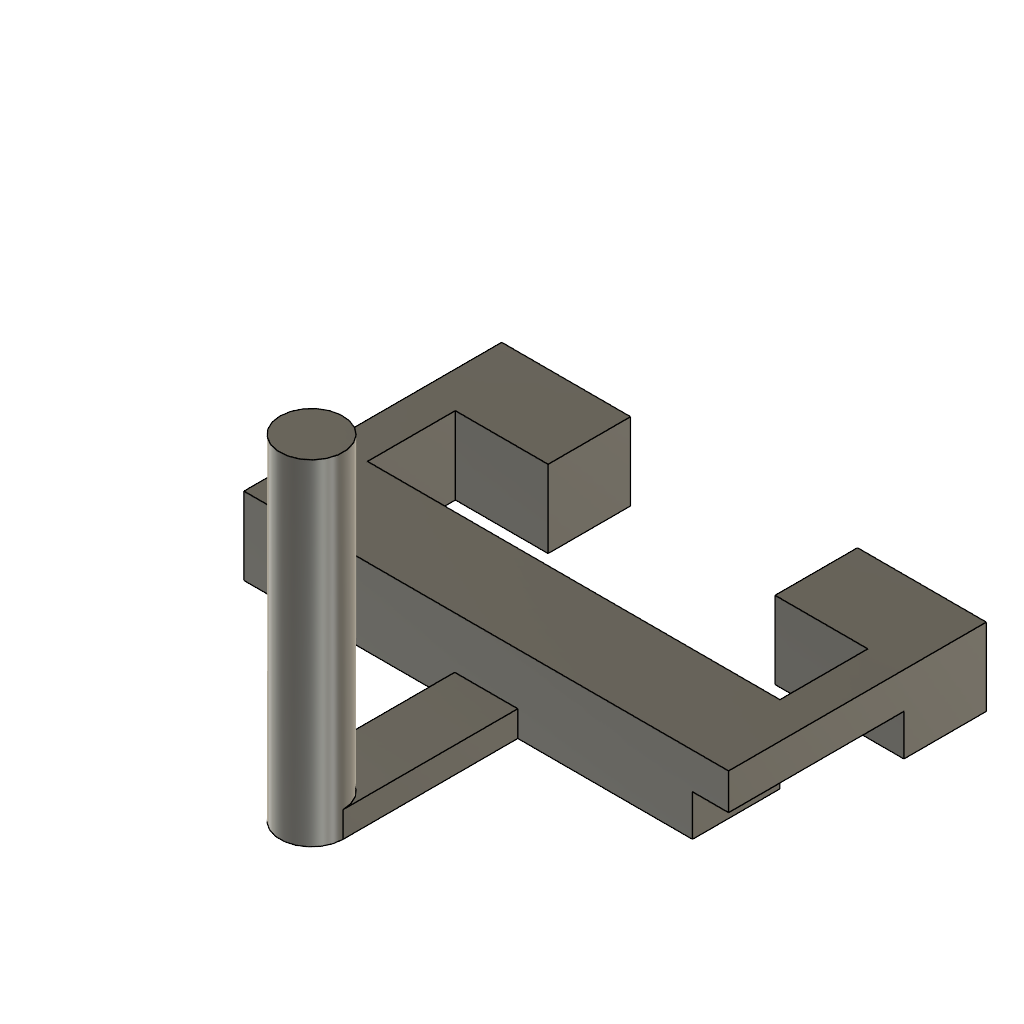
Bracket_Design_A6 (Autodesk Fusion 360 design; units mm, degrees)
part number: 2026-09-29-19-47-02-851
Autodesk Fusion 360 part; units mm, degrees
note: some values were not read from the file. Chosen so that the rebuilt part matches the saved one: that a step has no effect. Set by a fixed rule: which sketch regions a step uses.
sketch "Sketch1" plane through (0, 0, 0) normal (0, 0, 1) x (1, 0, 0)
  circle A0 centre (0, 0) radius 7.772
  line L0 (-7.772, -7.772) -> (7.772, -7.772)
  line L1 (7.772, -7.772) -> (7.772, 43.028)
  line L2 (7.772, 43.028) -> (-7.772, 43.028)
  line L3 (-7.772, 43.028) -> (-7.772, -7.772)
  dimension "d31" = 15.5439
  dimension "d36" = 15.5439
  dimension "d37" = 50.8
  constraint coincident A0.centre origin
  constraint horizontal L0
  constraint vertical L1
  constraint horizontal L2
  constraint vertical L3
  constraint tangent A0 L3
  constraint tangent A0 L0
  measures "d31" diameter of A0
  measures "d36" distance of L0.start L0.end
  measures "d37" distance of L0.start L2.end
extrude "Extrude1" add sketch "Sketch1" along normal blind 76.2 contours A0
extrude "Extrude2" add sketch "Sketch1" against normal blind 6.35
extrude "Extrude3" cut sketch "Sketch1" against normal blind 10.16 contours A0 L0 L1 | A0 L0 L3
sketch "Sketch2" plane through (0, 0, 0) normal (0, 0, 1) x (1, 0, 0)
  line L0 (-50.8, 43.0276) -> (50.8, 43.0276)
  line L1 (50.8, 43.0276) -> (50.8, 64.5802)
  line L2 (50.8, 64.5802) -> (-50.8, 64.5802)
  line L3 (-50.8, 64.5802) -> (-50.8, 43.0276)
  dimension "d42" = 101.6
  dimension "d43" = 21.5526
  constraint horizontal L0
  constraint vertical L1
  constraint horizontal L2
  constraint vertical L3
  measures "d42" distance of L0.start L0.end
  measures "d43" distance of L0.start L2.end
extrude "Extrude4" add sketch "Sketch2" along normal blind 12.7
extrude "Extrude5" add 1 faces at (-2.5907, 57.3962, 0) along direction (0, 0, -1) blind 6.35
sketch "Sketch3" plane through (50.8, 0, 0) normal (1, 0, 0) x (0, 1, 0)
  line L0 (64.5802, -6.35) -> (64.5802, 12.7)
  line L1 (64.5802, 12.7) -> (43.0276, 12.7)
  line L2 (43.0276, 12.7) -> (43.0276, -6.35)
  line L3 (43.0276, -6.35) -> (64.5802, -6.35)
  line L4 (43.0276, 0) -> (43.0276, -6.35)
  line L5 (43.0276, -6.35) -> (43.0276, 12.7)
  line L6 (43.0276, 12.7) -> (43.0276, -6.35)
  line L7 (43.0276, -6.35) -> (43.0276, 0)
  line L8 (43.0276, 12.7) -> (106.5276, 12.7)
  line L9 (106.5276, 12.7) -> (106.5276, 3.81)
  line L10 (106.5276, 3.81) -> (43.0276, 3.81)
  line L11 (43.0276, 3.81) -> (43.0276, 12.7)
  dimension "d48" = 63.5
  constraint horizontal L8
  constraint vertical L9
  constraint horizontal L10
  constraint vertical L11
  constraint coincident L1.end L2.start
  measures "d48" distance of L1.end L8.end
sketch "Sketch4" plane through (-50.8, 0, 0) normal (-1, 0, 0) x (0, -1, 0)
  line L0 (-43.0276, -6.35) -> (-43.0276, 12.7)
  line L1 (-43.0276, 12.7) -> (-64.5802, 12.7)
  line L2 (-64.5802, 12.7) -> (-64.5802, -6.35)
  line L3 (-64.5802, -6.35) -> (-43.0276, -6.35)
  line L4 (-43.0276, 12.7) -> (-106.5276, 12.7)
  line L5 (-106.5276, 12.7) -> (-106.5276, -6.3787)
  line L6 (-106.5276, -6.3787) -> (-43.0276, -6.3787)
  line L7 (-43.0276, -6.3787) -> (-43.0276, 12.7)
  dimension "d49" = 63.5
  constraint horizontal L4
  constraint vertical L5
  constraint horizontal L6
  constraint vertical L7
  constraint coincident L0.end L1.start
  measures "d49" distance of L0.end L4.end
extrude "Extrude6" add sketch "Sketch4" along normal blind 8.89
extrude "Extrude7" add sketch "Sketch3" along normal blind 8.89 contours L0 L1 L2 L5 L6 L8 L10 L11 | L0 L8 L9 L10
sketch "Sketch5" plane through (0, 106.5276, 0) normal (0, 1, 0) x (-1, 0, 0)
  line L0 (-50.8, 3.81) -> (-50.8, 12.7)
  line L1 (-50.8, 12.7) -> (-59.69, 12.7)
  line L2 (-59.69, 12.7) -> (-59.69, 3.81)
  line L3 (-59.69, 3.81) -> (-50.8, 3.81)
  line L4 (-59.69, 12.7) -> (-27.94, 12.7)
  line L5 (-27.94, 12.7) -> (-27.94, -6.35)
  line L6 (-27.94, -6.35) -> (-59.69, -6.35)
  line L7 (-59.69, -6.35) -> (-59.69, 12.7)
  line L8 (59.69, 12.7) -> (27.94, 12.7)
  line L9 (27.94, 12.7) -> (27.94, -6.35)
  line L10 (27.94, -6.35) -> (59.69, -6.35)
  line L11 (59.69, -6.35) -> (59.69, 12.7)
  dimension "d54" = 31.75
  dimension "d55" = 19.05
  dimension "d56" = 31.75
  dimension "d57" = 19.05
  constraint horizontal L4
  constraint vertical L5
  constraint horizontal L6
  constraint vertical L7
  constraint coincident L1.end L2.start
  constraint horizontal L8
  constraint vertical L9
  constraint horizontal L10
  constraint vertical L11
  measures "d54" distance of L1.end L4.end
  measures "d55" distance of L1.end L6.end
  measures "d56" distance of L8.start L8.end
  measures "d57" distance of L8.start L10.end
extrude "Extrude8" add sketch "Sketch5" against normal blind 20.32
extrude "Extrude9" [no effect]
extrude "Extrude10" [no effect]
extrude "Extrude11" [no effect]
extrude "Extrude12" cut 1 faces at (-35.56, 99.7543, -6.35) along direction (0, 0, 1) blind 0.508
extrude "Extrude13" add 1 faces at (-35.56, 99.7543, -5.842) along direction (0, 0, -1) blind 0.508
extrude "Extrude14" [no effect]
extrude "Extrude15" add 1 faces at (-53.7633, 85.3609, -6.3787) along direction (0, 0, -1) blind 1.524
extrude "Extrude16" cut 1 faces at (-53.7633, 85.3609, -7.9027) along direction (0, 0, 1) blind 1.524
equation "Force = 600 lbforce"
equation "SF = 4.0"
equation "S_y = 40000 psi"
equation "Sigma_allow = S_y / SF"
equation "E_ = 10000000 psi"
equation "Delta_max = 0.005 in"
equation "L_A = 3 in"
equation "r_A = ( ( ( 4 * ( ( Force * L_A ) / 8 ) ) / ( PI * Sigma_allow ) ) / 1 in^3 ) ^ ( 1 / 3 ) * 1 in"
equation "D_A = 2 * r_A"
equation "L_B = 2 in"
equation "w_B = D_A"
equation "t_B = 0.250 in"
equation "A_B = w_B * t_B"
equation "L_C = 4 in"
equation "b_C = 0.5 in"
equation "M_max_C = ( Force * L_C ) / 4"
equation "Z_rec_C = ( ( Force * L_C ) / 4 ) / Sigma_allow"
equation "h_C = ( ( ( 6 * 0.06 ) / 0.5 ) ^ ( 1 / 2 ) ) * 1 in"
equation "P_D = Force / 2"
equation "L_D = 2.5 in"
equation "I_D_min = ( P_D * ( L_D * L_D * L_D ) ) / ( 3 * E_ * Delta_max )"
equation "t_D = 0.350 in"
equation "P_E = Force / 2"
equation "L_E = 2 in"
equation "I_E_min = 0.0160"
equation "b_f = 1.250 in"
equation "t_f = 0.200 in"
equation "h_s = 0.8 in"
equation "t_s = 0.2 in"
equation "d31 = D_A"
equation "d36 = w_B"
equation "d37 = L_B"
equation "d42 = L_C"
equation "d43 = h_C"
equation "d44 = b_C"
equation "d48 = L_D"
equation "d49 = L_D"
